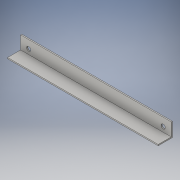
# Autodesk Inventor part: Side bar1
Saved by Autodesk Inventor 2016 (Build 200138000, 138)
## iProperties
Created: 2017-11-01
Part Number: Side bar1
Material: Generic
Document SubType Name: Modeling
Designer: thompson.nathaniel
Density: 1 g/cm^3
Appearance: Default
Author: thompson.nathaniel
Autodesk Inventor part; units mm, degrees
ref_plane "YZ Plane" through (0, 0, 0) normal (1, 0, 0) x (0, 1, 0)
ref_plane "XZ Plane" through (0, 0, 0) normal (0, 1, 0) x (-1, 0, 0)
ref_plane "XY Plane" through (0, 0, 0) normal (0, 0, 1) x (1, 0, 0)
sketch "Sketch1" plane through (0, 0, 0) normal (1, 0, 0) x (0, 1, 0)
  line L0 (3.175, 0) -> (3.175, -34.925)
  line L1 (3.175, -34.925) -> (38.1, -34.925)
  line L2 (38.1, -34.925) -> (38.1, -38.1)
  line L3 (38.1, -38.1) -> (0, -38.1)
  line L4 (0, -38.1) -> (0, 0)
  line L5 (0, 0) -> (3.175, 0)
  dimension "d0" = 3.175
  dimension "d1" = 3.175
  dimension "d2" = 38.1
  dimension "d3" = 38.1
  dimension "d4" = 0
  dimension "d5" = 0
  constraints: 12 end point, 5 perpendicular, 1 vertical
  measures "d0" distance of L4.end L0.start
  measures "d1" distance of L1.end L2.end
  measures "d2" distance of L3.end L4.end
  measures "d3" distance of L2.end L3.end
  measures "d4" distance from line of point (0, 0) L4
  measures "d5" distance from line of point (0, 0) L5
extrude "Extrusion1" add sketch "Sketch1" along normal blind 403.225
sketch "Sketch2" plane through (0, 3.175, -34.925) normal (0, 0, 1) x (1, 0, 0)
  circle A0 centre (21.59, 13.335) radius 5.715
  line L0 (0, -3.175) -> (403.225, -3.175) projected
  line L1 (403.225, 34.925) -> (403.225, 0) projected
  line L2 (0, 0) -> (0, 34.925) projected
  line L3 (0, 0) -> (403.225, 0) projected
  dimension "d10" = 11.43
  dimension "d13" = 21.59
  dimension "d19" = 13.335
  constraints: 1 centre point
  measures "d10" diameter of A0
  measures "d13" distance from line of L2 A0.centre
  measures "d19" distance from line of L3 A0.centre
extrude "Extrusion2" cut sketch "Sketch2" against normal blind 25.4
sketch "Sketch3" plane through (0, 3.175, -34.925) normal (0, 0, 1) x (1, 0, 0)
  circle A0 centre (381.635, 13.335) radius 5.715
  line L0 (403.225, 34.925) -> (403.225, 0) projected
  line L1 (0, 0) -> (403.225, 0) projected
  point P0 (0, -3.175)
  dimension "d14" = 11.43
  dimension "d15" = 21.59
  dimension "d16" = 13.335
  constraints: 1 centre point
  measures "d14" diameter of A0
  measures "d15" distance from line of L0 A0.centre
  measures "d16" distance from line of L1 A0.centre
extrude "Extrusion3" cut sketch "Sketch3" against normal blind 25.4
body "Solid1"
